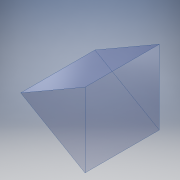
# Autodesk Inventor part: Prisma-12.7
Saved by Autodesk Inventor 2017 (Build 210142000, 142)
## iProperties
Created: 2017-08-01
Part Number: Prisma-12.7
Material: Glass
Document SubType Name: Modeling
Designer: vmiguel
Density: 2.18 g/cm^3
Appearance: Tropical Blue
Author: vmiguel
Autodesk Inventor part; units mm, degrees
ref_plane "YZ Plane" through (0, 0, 0) normal (1, 0, 0) x (0, 1, 0)
ref_plane "XZ Plane" through (0, 0, 0) normal (0, 1, 0) x (-1, 0, 0)
ref_plane "XY Plane" through (0, 0, 0) normal (0, 0, 1) x (1, 0, 0)
sketch "Sketch1" plane through (0, 0, 0) normal (0, 1, 0) x (-1, 0, 0)
  line L0 (-3.6662, -6.35) -> (-3.6662, 6.35)
  line L1 (-3.6662, 6.35) -> (7.3323, 0)
  line L2 (7.3323, 0) -> (-3.6662, -6.35)
  point P0 (0, 0)
  point P1 (0, 0)
  point P2 (-3.6662, 0)
  dimension "d0" = 12.7
  constraints: 6 end point, 1 coincident, 1 horizontal alignment, 1 midpoint, 7 other
  measures "d0" distance of L0.end L1.end
extrude "Extrusion1" add sketch "Sketch1" along normal blind 12.7
body "Solid1"
